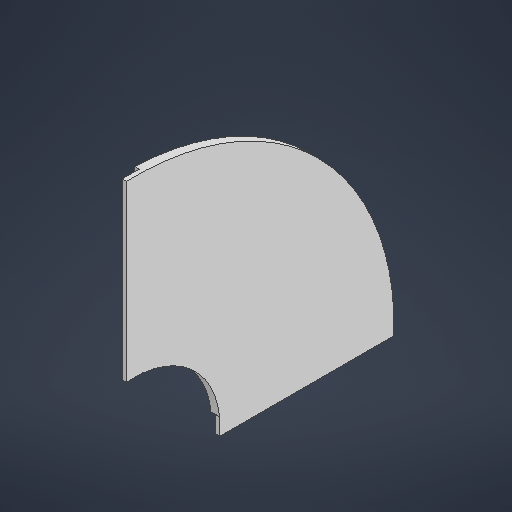
# Autodesk Inventor part: Part1
Saved by Autodesk Inventor 2026.2 (Build 302298000, 298)
## iProperties
Created: 2025-12-09
Part Number: Part1
Material: Generic
Document SubType Name: Modeling
Designer: Thoma
Density: 1 g/cm^3
Appearance: Default
Author: Thoma
Autodesk Inventor part; units mm, degrees
ref_plane "YZ Plane" through (0, 0, 0) normal (1, 0, 0) x (0, 1, 0)
ref_plane "XZ Plane" through (0, 0, 0) normal (0, 1, 0) x (-1, 0, 0)
ref_plane "XY Plane" through (0, 0, 0) normal (0, 0, 1) x (1, 0, 0)
sketch "Sketch1" plane through (0, 0, 0) normal (1, 0, 0) x (0, 1, 0)
  line L0 (152.4, 0) -> (152.4, -152.4)
  line L1 (152.4, -152.4) -> (0, -152.4)
  circle A0 centre (0, 0) radius 152.4
  arc A1 (0, -152.4) -> (152.4, 0) centre (0, 0) ccw
  line L2 (152.318, 5) -> (50, 5)
  line L3 (50, -5) -> (50, 5)
  line L4 (152.318, -5) -> (49.7494, -5)
  line L5 (5, -49.7494) -> (5, -152.318)
  line L6 (-5, -50) -> (-5, -152.318)
  line L7 (5, -50) -> (-5, -50)
  arc A2 (50, 0) -> (0, -50) centre (0, 0) ccw
  arc A3 (5, -49.7494) -> (49.7494, -5) centre (0, 0) ccw
  dimension "d7" = 152.4
  dimension "d8" = 50
  dimension "d9" = 50
  dimension "d10" = 147.4
  dimension "d11" = 157.4
  dimension "d12" = 10
  dimension "d13" = 157.4
  dimension "d14" = 147.4
  constraints: 16 end point, 11 point on circle, 4 centre point, 4 tangent, 3 parallel, 3 vertical, 2 coincident, 2 midpoint, 1 concentric, 1 horizontal, 1 perpendicular, 1 point on line
  measures "d7" radius of A1
  measures "d8" radius of A3
  measures "d9" radius of A2
  measures "d10" distance between parallel lines of L0 L5
  measures "d11" distance between parallel lines of L0 L6
  measures "d12" distance between parallel lines of L2 L4
  measures "d13" distance between parallel lines of L1 L2
  measures "d14" distance from line of L7.start L0
extrude "Extrusion1" add sketch "Sketch1" along normal blind 5 contours A0 L5 A3 L4
sketch "Sketch2" plane through (5, 0, 0) normal (1, 0, 0) x (0, 0, -1)
  line L0 (49.7494, 5) -> (152.318, 5) projected
  line L1 (50, 5) -> (50, -5)
  line L2 (0, 152.4) -> (0, 0)
  line L3 (5, 152.318) -> (5, 49.7494) projected
  line L4 (0, 0) -> (152.4, 0)
  arc A0 (152.4, 0) -> (0, 152.4) centre (0, 0) ccw
  arc A1 (152.318, 5) -> (5, 152.318) centre (0, 0) ccw projected
  line L5 (50, -5) -> (152.318, -5)
  arc A2 (152.318, -5) -> (152.318, 5) centre (0, 0) ccw
  line L6 (-5, 50) -> (5, 50)
  line L7 (5, 50) -> (5, 152.318)
  arc A3 (5, 152.318) -> (-5, 152.318) centre (0, 0) ccw
  line L8 (-5, 152.318) -> (-5, 50)
  arc A4 (49.7494, 5) -> (5, 49.7494) centre (0, 0) ccw
  arc A5 (0, 50) -> (50, 0) centre (0, 0) ccw
  point P0 (0, 152.4)
  dimension "d18" = 10
  dimension "d19" = 152.4
  dimension "d20" = 152.4
  dimension "d23" = 90
  dimension "d25" = 152.4
  constraints: 16 end point, 13 point on circle, 5 centre point, 2 horizontal, 2 midpoint, 2 parallel, 2 point on line, 2 tangent, 1 coincident, 1 perpendicular, 11 other
  measures "d18" distance of L1.end L1.start
  measures "d19" distance of L2.start L2.end
  measures "d20" distance of L2.end L4.end
  measures "d25" radius of A2
extrude "Extrusion2" add sketch "Sketch2" against normal blind 2.5 contours L0 A0 L4 L1 | L4 A2 L5 L1 | L6 L2 A0 L3 | L6 L8 A3 L2
body "Solid1"
